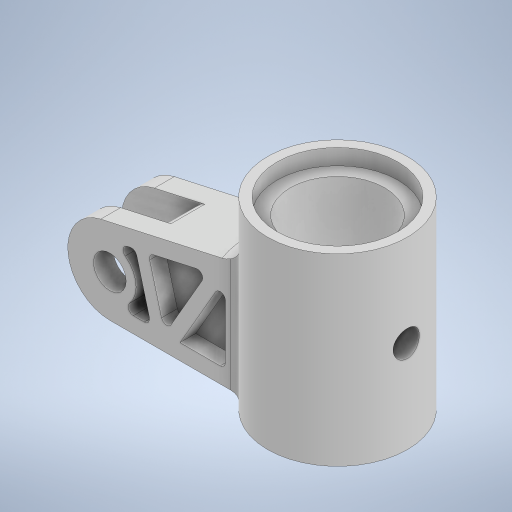
# Autodesk Inventor part: External_roller
Saved by Autodesk Inventor 2023 (Build 270158000, 158)
## iProperties
Created: 2024-07-20
Part Number: External_roller
Material: Generic
Document SubType Name: Modeling
Designer: plebbb
Density: 1 g/cm^3
Appearance: Default
Author: plebbb
Autodesk Inventor part; units mm, degrees
ref_plane "XZ Plane" through (0, 0, 0) normal (0, 1, 0) x (-1, 0, 0)
sketch "Sketch1" plane through (0, 0, 0) normal (1, 0, 0) x (0, 1, 0)
  line L0 (3, 9) -> (32, 9)
  line L1 (32, 9) -> (32, 11.5)
  line L2 (32, 11.5) -> (35, 11.5)
  line L3 (35, 11.5) -> (35, 13.3)
  line L4 (35, 13.3) -> (0, 13.3)
  line L5 (0, 13.3) -> (0, 11.5)
  line L6 (0, 11.5) -> (3, 11.5)
  line L7 (3, 11.5) -> (3, 9)
  line L8 (-7, 0) -> (42, 0) projected
  point P0 (0, 0)
  dimension "d0" = 1.8
  dimension "d1" = 2.5
  dimension "d2" = 11.5
  dimension "d3" = 3
  dimension "d4" = 35
  constraints: 16 end point, 7 perpendicular, 2 equal length, 1 horizontal, 1 vertical alignment
  measures "d0" distance of L2.end L3.end
  measures "d1" distance of L0.end L1.end
  measures "d2" distance of point (0, 0) L5.end
  measures "d3" distance of L1.end L2.end
  measures "d4" distance of L3.end L4.end
revolve "Revolution1" add sketch "Sketch1" angle 360 about axis through (0, -10, 0) along (0, 1, 0)
ref_plane "Work Plane1" through (13.3, 17.5, 0) normal (1, 0, 0) x (0, 1, 0)
sketch "Sketch2" plane through (13.3, 17.5, 0) normal (1, 0, 0) x (0, 1, 0)
  circle A0 centre (0, 0) radius 2.5
  line L0 (-17.5, -13.3) -> (-17.5, 13.3) projected
  point P0 (-17.5, 0)
  dimension "d6" = 17.5
  dimension "d7" = 5
  constraints: 1 centre point, 1 horizontal alignment
  measures "d6" distance from line of L0 A0.centre
  measures "d7" diameter of A0
extrude "Extrusion1" cut sketch "Sketch2" against normal up to surface
ref_plane "Work Plane6" through (0, 0, 7) normal (0, 0, 1) x (1, 0, 0)
sketch "Sketch6" plane through (0, 0, 7) normal (0, 0, 1) x (1, 0, 0)
  line L0 (-11.3088, 35) -> (-11.3088, 0)
  line L1 (-11.3088, 0) -> (-36.3088, 0)
  arc A0 (-38.0404, 15.8104) -> (-36.3088, 0) centre (-36.3088, 8) ccw
  line L2 (-38.0404, 15.8104) -> (-11.3088, 21.7366)
  point P0 (0, 0)
  dimension "d19" = 8
  dimension "d20" = 25
  dimension "d21" = 12.5
  constraints: 6 end point, 2 coincident, 2 point on circle, 2 tangent, 1 centre point, 1 horizontal, 1 point on line
  measures "d19" radius of A0
  measures "d20" distance from line of L0 A0.centre
  measures "d21" angle of L1 L2
extrude "Extrusion3" add sketch "Sketch6" against normal blind 14
sketch "Sketch8" plane through (0, 0, -7) normal (0, 0, -1) x (-1, 0, 0)
  arc A0 (36.3088, 0) -> (38.0404, 15.8104) centre (36.3088, 8) ccw projected
  circle A1 centre (36.3088, 8) radius 3.1115
  point P0 (0, 0)
  dimension "d35" = 6.223
  constraints: 1 centre point, 1 coincident
  measures "d35" diameter of A1
extrude "Extrusion5" cut sketch "Sketch8" against normal up to next
sketch "Sketch9" plane through (0, 0, 0) normal (0, 0, 1) x (1, 0, 0)
  circle A0 centre (-36.3088, 8) radius 3.1115 projected
  arc A1 (-38.0404, 15.8104) -> (-36.3088, 0) centre (-36.3088, 8) ccw projected
  circle A2 centre (-36.3088, 8) radius 9.5
  point P0 (0, 0)
  dimension "d38" = 19
  constraints: 1 centre point, 1 coincident
  measures "d38" diameter of A2
extrude "Extrusion6" cut sketch "Sketch9" along normal mid plane 6.45 contours A0 | A2
fillet "Fillet2" radius 2 2 edges at (-33.0383, 16.9193, 0) (-31.1854, 0, 0)
sketch "Sketch7" plane through (0, 0, -7) normal (0, 0, -1) x (-1, 0, 0)
  line L0 (14.3088, 17.9987) -> (37.391, 12.8815)
  circle A0 centre (36.3088, 8) radius 5
  line L1 (36.3088, 3) -> (14.3088, 3)
  line L2 (14.3088, 3) -> (14.3088, 17.9987)
  line L3 (11.3088, 0) -> (11.3088, 21.7366) projected
  line L4 (11.3088, 0) -> (36.3088, 0) projected
  arc A1 (36.3088, 0) -> (38.0404, 15.8104) centre (36.3088, 8) ccw projected
  line L5 (38.0404, 15.8104) -> (11.3088, 21.7366) projected
  line L6 (14.3088, 17.9987) -> (22.9683, 3)
  line L7 (25.8551, 3) -> (17.6193, 17.2648)
  line L8 (25.8551, 3) -> (29.0012, 14.7415)
  line L9 (31.4443, 14.1998) -> (28.4433, 3)
  line L10 (19.5721, 8.8824) -> (21.7372, 10.1324) construction
  line L11 (27.4281, 8.8707) -> (29.843, 8.2237) construction
  arc A2 (33.3919, 12.0609) -> (33.0249, 13.8494) centre (32.8085, 12.8731) ccw
  arc A3 (31.8367, 3) -> (32.5821, 4.6667) centre (31.8367, 4) ccw
  point P0 (0, 0)
  dimension "d24" = 3
  dimension "d25" = 3
  dimension "d27" = 2.5
  dimension "d28" = 30
  dimension "d30" = 45
  dimension "d31" = 1
  constraints: 18 end point, 10 point on line, 8 point on circle, 6 tangent, 4 parallel, 3 centre point, 2 midpoint, 2 perpendicular, 1 coincident, 1 equal length, 1 equal radius, 1 vertical
  measures "d24" radial gap between concentric circles of A1 A0
  measures "d25" distance between parallel lines of L3 L2
  measures "d27" distance of L10.start L10.end
  measures "d28" angle of L2 L6
  measures "d30" angle of L7 L8
  measures "d31" radius of A2
extrude "Extrusion4" cut sketch "Sketch7" against normal blind 3 contours L6 L1 L2 | L0 L8 L7 | L0 A2 A0 A3 L1 L9
fillet "Fillet1" radius 1 7 edges at (-14.3088, 3, -5.5) (-14.3088, 17.9987, -5.5) (-17.6193, 17.2648, -5.5) (-29.0012, 14.7415, -5.5) (-25.8551, 3, -5.5) (-28.4433, 3, -5.5) (-31.4443, 14.1998, -5.5)
fillet "Fillet3" radius 4 3 edges at (-11.3088, 10.8683, -7) (-13.3, 21.2952, 0) (-11.3088, 10.8683, 7)
mirror "Mirror1" about plane through (0, 0, 0) normal (0, 0, 1) of "Extrusion4", "Fillet1"
body "Solid1"
